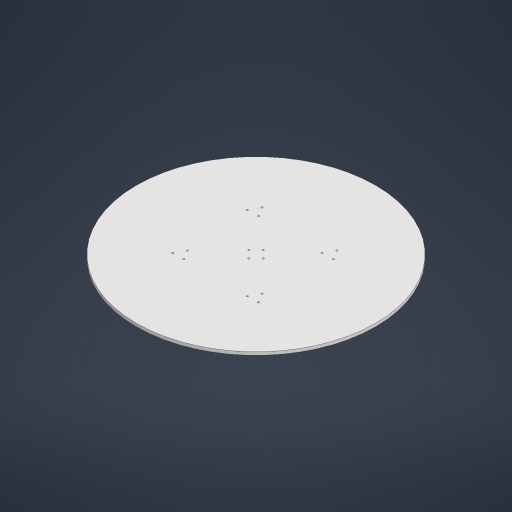
# Autodesk Inventor part: Base
Saved by Autodesk Inventor 2023 (Build 270158000, 158)
## iProperties
Created: 2023-10-25
Part Number: Base
Material: Generic
Document SubType Name: Modeling
Designer: Abhinav
Density: 1 g/cm^3
Appearance: Default
Author: Abhinav
Autodesk Inventor part; units mm, degrees
ref_plane "YZ Plane" through (0, 0, 0) normal (1, 0, 0) x (0, 1, 0)
ref_plane "XZ Plane" through (0, 0, 0) normal (0, 1, 0) x (-1, 0, 0)
ref_plane "XY Plane" through (0, 0, 0) normal (0, 0, 1) x (1, 0, 0)
sketch "Sketch1" plane through (0, 0, 0) normal (0, 1, 0) x (-1, 0, 0)
  circle A0 centre (0, 0) radius 200
  circle A1 centre (-62.1988, 52) radius 1.5
  circle A2 centre (-71.7439, 67.4891) radius 1.5
  circle A3 centre (-62.5, 62.5) radius 13.5 construction
  circle A4 centre (-53.5573, 68.0109) radius 1.5
  circle A5 centre (53.2561, 67.4891) radius 1.5
  circle A6 centre (62.8012, 52) radius 1.5
  circle A7 centre (71.4427, 68.0109) radius 1.5
  circle A8 centre (62.5, 62.5) radius 13.5 construction
  circle A9 centre (53.2561, -57.5109) radius 1.5
  circle A10 centre (62.8012, -73) radius 1.5
  circle A11 centre (71.4427, -56.9891) radius 1.5
  circle A12 centre (62.5, -62.5) radius 13.5 construction
  circle A13 centre (-71.7439, -57.5109) radius 1.5
  circle A14 centre (-62.1988, -73) radius 1.5
  circle A15 centre (-53.5573, -56.9891) radius 1.5
  circle A16 centre (-62.5, -62.5) radius 13.5 construction
  line L0 (-62.5, 62.5) -> (62.5, 62.5)
  line L1 (62.5, 62.5) -> (62.5, -62.5)
  line L2 (62.5, -62.5) -> (-62.5, -62.5)
  line L3 (-62.5, -62.5) -> (-62.5, 62.5)
  line L4 (-62.5, 62.5) -> (62.5, -62.5) construction
  line L5 (62.5, 62.5) -> (-62.5, -62.5) construction
  circle A17 centre (0, 0) radius 15 construction
  circle A18 centre (0, 0) radius 4 construction
  line L6 (0, 0) -> (-12, 0) construction
  line L7 (0, 0) -> (0, -12) construction
  circle A19 centre (0, -12) radius 1.5
  circle A20 centre (-12, 0) radius 1.5
  circle A21 centre (12, 0) radius 1.5
  circle A22 centre (0, 12) radius 1.5
  point P0 (-62.5, 62.5)
  point P1 (-62.5, 62.5)
  point P2 (-62.5, 62.5)
  point P3 (62.5, 62.5)
  point P4 (62.5, 62.5)
  point P5 (62.5, 62.5)
  point P6 (62.5, -62.5)
  point P7 (62.5, -62.5)
  point P8 (62.5, -62.5)
  point P9 (-62.5, -62.5)
  point P10 (-62.5, -62.5)
  point P11 (-62.5, -62.5)
  dimension "d0" = 400
  dimension "d5" = 125
  dimension "d6" = 30
  dimension "d7" = 8
  dimension "d8" = 12
  dimension "d9" = 12
  dimension "d10" = 3
  dimension "d11" = 3
  constraints: 23 centre point, 16 end point, 4 coincident, 2 horizontal, 2 midpoint, 2 parallel, 2 perpendicular, 2 symmetric about line, 1 vertical, 3 other
  measures "d0" diameter of A0
  measures "d5" distance of L0.end L1.end
  measures "d6" diameter of A17
  measures "d7" diameter of A18
  measures "d8" distance of L6.start L6.end
  measures "d9" distance of L6.start L7.end
  measures "d10" diameter of A19
  measures "d11" diameter of A20
extrude "Extrusion1" add sketch "Sketch1" along normal blind 5 contours A0 | A1 L3 L0 L1 A6 L2
body "Solid1"
